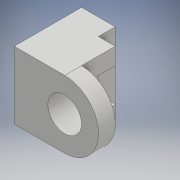
# Autodesk Inventor part: 34
Saved by Autodesk Inventor 2017 (Build 210142000, 142)
## iProperties
Part Number: 34
Material: 一般
Document SubType Name: Modeling
Designer: Brian
Density: 1 g/cm^3
Appearance: 預設
Author: Brian
Autodesk Inventor part; units mm, degrees
ref_plane "YZ Plane" through (0, 0, 0) normal (1, 0, 0) x (0, 1, 0)
ref_plane "XZ Plane" through (0, 0, 0) normal (0, 1, 0) x (-1, 0, 0)
ref_plane "XY Plane" through (0, 0, 0) normal (0, 0, 1) x (1, 0, 0)
sketch "草圖1" plane through (0, 0, 0) normal (0, 0, 1) x (1, 0, 0)
  line L0 (0, 0) -> (50, 0)
  line L1 (50, 0) -> (50, 10)
  line L2 (50, 10) -> (0, 10)
  line L3 (0, 10) -> (0, 0)
  line L4 (0, 10) -> (30, 10)
  line L5 (30, 10) -> (30, 30)
  line L6 (30, 30) -> (0, 30)
  line L7 (0, 30) -> (0, 10)
  line L8 (0, 30) -> (20, 30)
  line L9 (20, 30) -> (20, 40)
  line L10 (20, 40) -> (0, 40)
  line L11 (0, 40) -> (0, 30)
  dimension "d0" = 20
  dimension "d1" = 30
  dimension "d2" = 50
  dimension "d3" = 10
  dimension "d4" = 10
  dimension "d5" = 20
  constraints: 24 end point, 6 parallel, 3 horizontal, 3 perpendicular
  measures "d0" distance of L9.end L10.end
  measures "d1" distance of L5.end L6.end
  measures "d2" distance of L1.end L2.end
  measures "d3" distance of L2.end L0.start
  measures "d4" distance of L8.end L9.end
  measures "d5" distance of L4.end L5.end
extrude "擠出1" add sketch "草圖1" against normal blind 40
fillet "圓角1" radius 20 2 edges at (50, 5, 0) (50, 5, -40)
hole "孔1" at (30, 0, -20) direction (0, 1, 0) diameter 20 depth 50 tip angle 118
